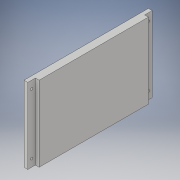
# Autodesk Inventor part: BatteryHighFront
Saved by Autodesk Inventor 2019 (Build 230136000, 136)
## iProperties
Created: 2017-11-10
Part Number: BatteryHighFront
Material: Generic
Document SubType Name: Modeling
Designer: james
Density: 1 g/cm^3
Appearance: Default
Author: james
Autodesk Inventor part; units mm, degrees
ref_plane "YZ Plane" through (0, 0, 0) normal (1, 0, 0) x (0, 1, 0)
ref_plane "XZ Plane" through (0, 0, 0) normal (0, 1, 0) x (-1, 0, 0)
ref_plane "XY Plane" through (0, 0, 0) normal (0, 0, 1) x (1, 0, 0)
sketch "Sketch1" plane through (0, 0, 0) normal (0, 1, 0) x (-1, 0, 0)
  line L0 (10.1865, 69.048) -> (10.1865, -140.502)
  line L1 (10.1865, -140.502) -> (3.8365, -140.502)
  line L2 (3.8365, -140.502) -> (3.8365, -127.802)
  line L3 (3.8365, -127.802) -> (-2.5135, -127.802)
  line L4 (-2.5135, -127.802) -> (-2.5135, 56.348)
  line L5 (-2.5135, 56.348) -> (3.8365, 56.348)
  line L6 (3.8365, 56.348) -> (3.8365, 69.048)
  line L7 (3.8365, 69.048) -> (10.1865, 69.048)
  point P0 (0, 0)
  dimension "d0" = 184.15
  dimension "d1" = 6.35
  dimension "d2" = 6.35
  dimension "d3" = 12.7
  dimension "d4" = 12.7
  dimension "d5" = 6.35
  constraints: 16 end point, 7 perpendicular, 1 vertical
  measures "d0" distance of L3.end L4.end
  measures "d1" distance of L2.end L3.end
  measures "d2" distance of L0.end L1.end
  measures "d3" distance of L1.end L2.end
  measures "d4" distance of L5.end L6.end
  measures "d5" distance of L6.end L0.start
extrude "Extrusion1" add sketch "Sketch1" along normal blind 127
sketch "Sketch2" plane through (-3.8365, 0, 69.048) normal (1, 0, 0) x (0, 0, -1)
  line L0 (12.7, 0) -> (0, 0) projected
  line L1 (0, 0) -> (0, 127) projected
  line L2 (0, 127) -> (12.7, 127) projected
  point P0 (69.048, 0)
  point P1 (6.35, 114.3)
  point P2 (6.35, 12.7)
  dimension "d8" = 12.7
  dimension "d9" = 6.35
  dimension "d10" = 6.35
  dimension "d11" = 12.7
  measures "d8" distance from line of L0 point (6.35, 12.7)
  measures "d9" distance from line of L1 point (6.35, 12.7)
  measures "d10" distance from line of L1 point (6.35, 114.3)
  measures "d11" distance from line of L2 point (6.35, 114.3)
hole "Hole1" at (-3.8365, 114.3, 62.698) at (-3.8365, 12.7, 62.698) direction (-1, 0, 0) diameter 4.0386 depth 25.4 tip angle 118
sketch "Sketch3" plane through (-3.8365, 0, -127.802) normal (1, 0, 0) x (0, 0, -1)
  line L0 (12.7, 0) -> (0, 0) projected
  line L1 (12.7, 0) -> (12.7, 127) projected
  line L2 (12.7, 127) -> (-196.85, 127) projected
  point P0 (-127.802, 0)
  point P1 (6.35, 114.3)
  point P2 (6.35, 12.7)
  dimension "d19" = 12.7
  dimension "d20" = 6.35
  dimension "d21" = 6.35
  dimension "d22" = 12.7
  measures "d19" distance from line of L0 point (6.35, 12.7)
  measures "d20" distance from line of L1 point (6.35, 12.7)
  measures "d21" distance from line of L1 point (6.35, 114.3)
  measures "d22" distance from line of L2 point (6.35, 114.3)
hole "Hole2" at (-3.8365, 114.3, -134.152) at (-3.8365, 12.7, -134.152) direction (-1, 0, 0) diameter 4.0386 depth 25.4 tip angle 118
sketch "Sketch4" plane through (-10.1865, 0, -140.502) normal (-1, 0, 0) x (0, 0, 1)
  line L0 (25.4, 120.65) -> (184.15, 120.65)
  line L1 (184.15, 120.65) -> (184.15, 6.35)
  line L2 (184.15, 6.35) -> (25.4, 6.35)
  line L3 (25.4, 6.35) -> (25.4, 120.65)
  line L4 (196.85, 127) -> (12.7, 127) projected
  line L5 (209.55, 0) -> (0, 0) projected
  line L6 (0, 0) -> (0, 127) projected
  line L7 (209.55, 0) -> (209.55, 127) projected
  point P0 (140.502, 0)
  dimension "d30" = 6.35
  dimension "d31" = 6.35
  dimension "d32" = 25.4
  dimension "d33" = 25.4
  constraints: 8 end point, 2 parallel, 1 horizontal, 1 perpendicular
  measures "d30" distance between parallel lines of L4 L0
  measures "d31" distance between parallel lines of L5 L2
  measures "d32" distance between parallel lines of L6 L3
  measures "d33" distance between parallel lines of L7 L1
extrude "Extrusion2" cut sketch "Sketch4" against normal blind 3.175
sketch "Sketch5" plane through (0, 0, 0) normal (0, -1, 0) x (1, 0, 0)
  line L0 (2.5135, -127.802) -> (2.5135, 56.348) projected
  line L1 (-10.1865, -140.502) -> (-3.8365, -140.502) projected
  line L2 (-3.8365, 69.048) -> (-10.1865, 69.048) projected
  point P0 (0, 0)
  point P1 (-3.8365, -77.002)
  point P2 (-3.8365, 5.548)
  dimension "d36" = 6.35
  dimension "d37" = 6.35
  dimension "d38" = 63.5
  dimension "d39" = 63.5
  measures "d36" distance from line of L0 point (-3.836, 5.548)
  measures "d37" distance from line of L0 point (-3.836, -77.002)
  measures "d38" distance from line of L1 point (-3.836, -77.002)
  measures "d39" distance from line of L2 point (-3.836, 5.548)
hole "Hole3" at (-3.8365, 0, -77.002) at (-3.8365, 0, 5.548) direction (0, 1, 0) diameter 4.0386 depth 12.7 tip angle 118
body "Solid1"
